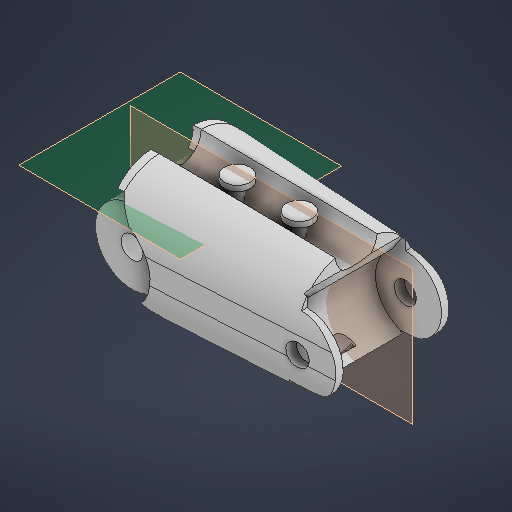
# Autodesk Inventor part: falange2_menique_V13
Saved by Autodesk Inventor 2026.1 (Build 301233020, 233B)
## iProperties
Created: 2026-01-14
Part Number: falange2_menique_V13
Material: Generic
Document SubType Name: Modeling
Designer: user
Density: 1 g/cm^3
Appearance: Default
Author: user
Autodesk Inventor part; units mm, degrees
ref_plane "YZ Plane" through (0, 0, 0) normal (1, 0, 0) x (0, 1, 0)
ref_plane "XY Plane" through (0, 0, 0) normal (0, 0, 1) x (1, 0, 0)
sketch "Sketch1" plane through (0, 0, 0) normal (0, 0, 1) x (1, 0, 0)
  line L0 (5.2681, -7.5236) -> (19.7319, -7.5236)
  circle A0 centre (0, 0) radius 1.5
  line L1 (0, 5) -> (0, 9.2)
  circle A1 centre (24, 0) radius 1.5
  arc A2 (21.8855, -4.448) -> (24, 4.925) centre (24, 0) ccw
  line L2 (24, 4.925) -> (24, 9.075)
  line L3 (24, 9.075) -> (0, 9.2)
  arc A3 (0, 5) -> (2.8679, -4.0958) centre (0, 0) ccw
  line L4 (2.8679, -4.0958) -> (5.2681, -7.5236)
  line L5 (21.8855, -4.448) -> (19.7319, -7.5236)
  dimension "d13" = 3
  dimension "d36" = 3
  dimension "d37" = 9.85
  dimension "d65" = 0
  dimension "d66" = 24
  dimension "d67" = 4.15
  dimension "d73" = 10
  dimension "d112" = 4.2
  dimension "d144" = 55
  constraints: 12 end point, 4 centre point, 4 point on circle, 3 coincident, 2 vertical, 1 parallel
  measures "d13" diameter of A0
  measures "d36" diameter of A1
  measures "d37" diameter of A2
  measures "d65" vertical distance of point (0, 0) A1.centre
  measures "d66" distance of A1.centre point (0, 0)
  measures "d67" distance of L2.start L2.end
  measures "d73" diameter of A3
  measures "d112" distance of L1.start L1.end
  measures "d144" angle of L0 L4
extrude "Extrusion1" add sketch "Sketch1" along normal mid plane 23
sketch "Sketch4" plane through (0, 9.2, -11.5) normal (-1, 0, 0) x (0, 0, 1)
  circle A0 centre (11.5, -13.8108) radius 1.5
  point P0 (11.5, -9.2)
  dimension "d23" = 3
  constraints: 1 centre point
  measures "d23" diameter of A0
extrude "Extrusion4" cut sketch "Sketch4" against normal blind 22.5
sketch "Sketch7" plane through (0, 0, 0) normal (0, 0, 1) x (1, 0, 0)
  circle A0 centre (25, 0) radius 5.075
  point P0 (0, 0)
  dimension "d116" = 10.15
  constraints: 1 centre point, 1 coincident
  measures "d116" diameter of A0
extrude "Extrusion6" cut sketch "Sketch7" along normal mid plane 13.41
ref_plane "Work Plane4" through (0, 0, 0) normal (0, 0, 1) x (1, 0, 0)
sketch "Sketch14" plane through (0, 0, 0) normal (0, 0, 1) x (1, 0, 0)
  circle A0 centre (0, 0) radius 5
  dimension "d80" = 10
  constraints: 1 centre point, 1 coincident
  measures "d80" diameter of A0
extrude "Extrusion12" cut sketch "Sketch14" along normal mid plane 3.825
sketch "Sketch39" plane through (5.2681, -7.5236, 11.5) normal (0, -1, 0) x (1, 0, 0)
  line L0 (-5.2681, -11.5) -> (20.8531, -11.5)
  line L1 (-5.2681, -2) -> (-27.6718, -2)
  line L2 (-27.6718, -2) -> (-27.6718, -11.5)
  line L3 (-27.6718, -11.5) -> (-5.2681, -11.5)
  line L4 (40.588, -3.8483) -> (40.569, -11.5)
  line L5 (40.569, -11.5) -> (20.8531, -11.5)
  line L6 (-27.6718, -21) -> (-27.6718, -11.5)
  line L7 (-5.2681, -21) -> (-27.6718, -21)
  line L8 (40.588, -19.1517) -> (40.569, -11.5)
  line L9 (18.7319, 0) -> (-5.2681, 0) projected
  line L10 (-5.2681, -23) -> (18.7319, -23) projected
  line L11 (-3.7681, -23) -> (-6.7681, -23) projected
  line L12 (-5.2681, -2) -> (-5.2681, 0)
  line L13 (-5.2681, -21) -> (-5.2681, -23)
  line L14 (-41.5239, -11.5) -> (55.441, -11.5) projected
  line L15 (18.7319, -4.795) -> (18.7319, -18.205) projected
  line L16 (18.7319, -23) -> (18.7319, 0) projected
  line L17 (18.7319, -11.5) -> (18.7319, -3.5)
  line L18 (-5.2681, -21) -> (40.5855, -18.1341)
  line L19 (-5.2681, -2) -> (40.5855, -4.8659)
  point P0 (-4.1469, -11.0242)
  point P1 (-3.1099, -9.8168)
  point P2 (20.8531, -20)
  point P3 (18.7319, -19.5)
  dimension "d161" = 9.5
  dimension "d162" = -23.963
  dimension "d168" = 0
  dimension "d169" = 8
  constraints: 28 end point, 5 symmetric about line, 3 perpendicular, 3 point on line, 2 horizontal, 1 collinear, 1 midpoint, 1 parallel, 1 vertical
  measures "d161" distance of L0.start L1.start
  measures "d162" horizontal distance of point (-3.11, -9.817) L0.end
  measures "d168" distance between parallel lines of L14 L3
  measures "d169" distance of L17.start L17.end
extrude "Extrusion24" cut sketch "Sketch39" against normal blind 24 contours L3 L2 L1 L19 L16 L15 L0 | L0 L15 L16 L18 L7 L6 L3 | L15 L16 L19 L4 L5 L0 | L0 L5 L8 L18 L16 L15 keep common part
fillet "Fillet5" radius 6.7625 2 edges at (12.5, -7.5236, -8.7188) (12.5, -7.5236, 8.7188)
fillet "Fillet6" radius 6.7625 2 edges at (12, 9.1375, 8.75) (12, 9.1375, -8.75)
sketch "Sketch12" plane through (0, 0, 11.5) normal (0, 0, 1) x (1, 0, 0)
  circle A0 centre (0, 0) radius 1.5 projected
  circle A1 centre (0, 0) radius 5.075
  dimension "d74" = 10.15
  constraints: 1 centre point, 1 coincident
  measures "d74" diameter of A1
extrude "Extrusion10" cut sketch "Sketch12" against normal blind 4.945
sketch "Sketch13" plane through (0, 0, -11.5) normal (0, 0, -1) x (-1, 0, 0)
  circle A0 centre (0, 0) radius 5.075
  dimension "d77" = 10.15
  constraints: 1 centre point
  measures "d77" diameter of A0
extrude "Extrusion11" cut sketch "Sketch13" against normal blind 4.945
sketch "Sketch16" plane through (0, 0, 0) normal (0, 0, 1) x (1, 0, 0)
  circle A0 centre (0, 0) radius 1.5 projected
  line L0 (-1.9036, 2.4472) -> (1.1675, 2.8722)
  line L1 (1.1675, 2.8722) -> (3.0711, 0.425)
  line L2 (3.0711, 0.425) -> (1.9036, -2.4472)
  line L3 (1.9036, -2.4472) -> (-1.1675, -2.8722)
  line L4 (-1.1675, -2.8722) -> (-3.0711, -0.425)
  line L5 (-3.0711, -0.425) -> (-1.9036, 2.4472)
  dimension "d83" = 5.37
  constraints: 12 end point, 1 coincident, 13 other
  measures "d83" distance between parallel lines of L3 L0
extrude "Extrusion13" cut sketch "Sketch16" along normal mid plane 8.085 contours A0 | L0 L1 L2 L3 L4 L5
ref_plane "Work Plane1" through (0, 9.2, -11.5) normal (0, 1, 0) x (-1, 0, 0)
sketch "Sketch27" plane through (24, 4.925, -11.5) normal (1, 0, 0) x (0, 0, -1)
  line L0 (0, 4.15) -> (-23, 4.15) projected
  circle A0 centre (-11.5, 4.15) radius 2.8604
  point P0 (-11.5, -4.925)
  dimension "d117" = 5.7208
  constraints: 1 centre point, 1 midpoint
  measures "d117" diameter of A0
sketch "Sketch28" plane through (0, 9.2, 11.5) normal (0.0052083, 0.9999864, 0) x (0.9999864, -0.0052083, 0)
  line L0 (24.0003, 23) -> (24.0003, 0) projected
  line L1 (24.0003, 11.5) -> (-8.1187, 11.5)
  point P0 (0.0479, 11.5)
  constraints: 2 end point, 1 horizontal, 1 midpoint
sweep "Sweep1" cut profiles "Sketch27" path "Sketch28" path curves L1
ref_plane "Work Plane2" through (0, 6.3396, 0) normal (-0.0052083, -0.9999864, 0) x (0.9999864, -0.0052083, 0)
sketch "Sketch30" plane through (0, 6.3396, 0) normal (-0.0052083, -0.9999864, 0) x (0.9999864, -0.0052083, 0)
  line L0 (24.0068, 6.705) -> (24.0068, -6.705) projected
  line L1 (24.0068, 0) -> (7.7668, 0)
  circle A0 centre (7.7668, 0) radius 0.7321
  point P0 (0.033, 0)
  dimension "d122" = 16.24
  dimension "d123" = 1.4642
  constraints: 2 end point, 1 centre point, 1 coincident, 1 horizontal, 1 midpoint
  measures "d122" distance of L1.start L1.end
  measures "d123" diameter of A0
extrude "Extrusion19" add sketch "Sketch30" against normal blind 2.1075
sketch "Sketch31" plane through (7.7777, 8.4066, 0) normal (0.0052083, 0.9999864, 0) x (0.9999864, -0.0052083, 0)
  circle A0 centre (0, 0) radius 0.7321 projected
  circle A1 centre (0, 0) radius 1.774
  point P0 (-7.7338, 0)
  dimension "d126" = 3.548
  constraints: 1 centre point, 1 coincident
  measures "d126" diameter of A1
extrude "Extrusion20" add sketch "Sketch31" along normal up to surface (0.7528 mm away) contours A0 | A1
sketch "Sketch34" plane through (0, 6.3396, 0) normal (-0.0052083, -0.9999864, 0) x (0.9999864, -0.0052083, 0)
  ellipse E0 centre (23.9854, 0) end of major axis (23.9854, -2.8604) minor radius 0.0149 (23.9865, -2.8535) -> (23.9865, 2.8535) ccw projected
  ellipse E1 centre (-0.0149, 0) end of major axis (-0.0149, -2.8604) minor radius 0.0149 (-0.0149, -2.8604) -> (-0.0149, 2.8604) ccw projected
  line L0 (-0.0149, 0) -> (16.2251, 0)
  circle A0 centre (16.2251, 0) radius 0.7321
  point P0 (0.033, 0)
  point P1 (0, 2.8604)
  point P2 (0, -2.8604)
  point P3 (-25.0003, -2.8604)
  point P4 (-25.0003, 2.8604)
  dimension "d130" = 16.24
  dimension "d131" = 1.4642
  constraints: 2 end point, 1 centre point, 1 coincident, 1 horizontal, 2 other
  measures "d130" distance of L0.start L0.end
  measures "d131" diameter of A0
extrude "Extrusion21" add sketch "Sketch34" against normal blind 2.1075
sketch "Sketch35" plane through (16.2359, 8.3626, 0) normal (0.0052083, 0.9999864, 0) x (0.9999864, -0.0052083, 0)
  circle A0 centre (0, 0) radius 0.7321 projected
  circle A1 centre (0, 0) radius 1.774
  point P0 (-16.1921, 0)
  dimension "d134" = 3.548
  constraints: 1 centre point, 1 coincident
  measures "d134" diameter of A1
extrude "Extrusion22" add sketch "Sketch35" along normal up to surface (0.7528 mm away) contours A0 | A1
chamfer "Chamfer1" distance 2 angle 45 1 edges at (24, 4.9755, 0)
chamfer "Chamfer2" distance 2 angle 45 2 edges at (0, 5.075, -7.7596) (0, 5.075, 7.7596)
sketch "Sketch36" plane through (0, 5, -6.555) normal (-1, 0, 0) x (0, 0, 1)
  arc A0 (3.6946, 4.1987) -> (9.4154, 4.1987) centre (6.555, 4.2) ccw projected
  line L0 (14.2123, 2.075) -> (13.11, 2.075) projected
  line L1 (14.2119, 2.0754) -> (8.4697, 2.075)
  arc A1 (8.4697, 2.075) -> (9.4154, 4.2) centre (6.555, 4.2) ccw
  arc A2 (6.555, 1.3396) -> (9.4154, 4.2) centre (6.555, 4.2) ccw
  line L2 (6.555, 5.0268) -> (6.555, -0.0494)
  line L3 (-1.1019, 2.0754) -> (0, 2.075)
  line L4 (-1.1019, 2.0754) -> (4.6403, 2.075)
  arc A3 (3.6946, 4.2) -> (4.6403, 2.075) centre (6.555, 4.2) ccw
  line L5 (0, -10) -> (0, 0) projected
  line L6 (3.9417, -5) -> (10.0382, -5)
  ellipse E0 centre (3.8307, -2.5626) end of major axis (-2.9217, -1.9999) minor radius 6.7625 (3.6946, 4.1987) -> (-1.1023, 2.075) ccw projected
  ellipse E1 centre (9.2793, -2.5626) end of major axis (16.0317, -1.9999) minor radius 6.7625 (14.2123, 2.075) -> (9.4154, 4.1987) ccw projected
  point P0 (6.555, -5)
  point P1 (0, 2.075)
  point P2 (8.4697, 2.075)
  point P3 (0, 2.075)
  point P4 (4.6403, 2.075)
  point P5 (14.2124, 2.075)
  point P6 (3.6946, 4.1987)
  constraints: 8 end point, 7 point on circle, 3 centre point, 2 coincident, 2 concentric, 2 symmetric about line, 1 horizontal, 1 vertical, 8 other
revolve "Revolution1" add sketch "Sketch36" angle 7 about axis through (0, 0, -2.6133) along (0, 0, 1)
equation "\"d13\" = diametroDentroUnion"
equation "\"d36\" = diametroDentroUnion"
equation "\"d73\" = diametroFueraUnion"
equation "\"d80\" = diametroFueraUnion"
equation "\"d16\" = 135deg"
equation "\"d26\" = 135deg"
equation "\"d27\" = 135deg"
equation "\"d30\" = 135deg"
equation "\"d34\" = 23"
equation "\"d35\" = 0"
equation "\"d40\" = 135deg"
equation "\"d41\" = 10.639"
equation "\"d42\" = 11.8875"
equation "\"d43\" = 0"
equation "\"diametroDentroUnion\" = 3"
equation "\"diametroFueraUnion\" = 10"
equation "\"d45\" = 15"
equation "\"d39\" = diametroDentroUnion"
equation "\"tolerancia\" = 0.15"
body "Solid1"
